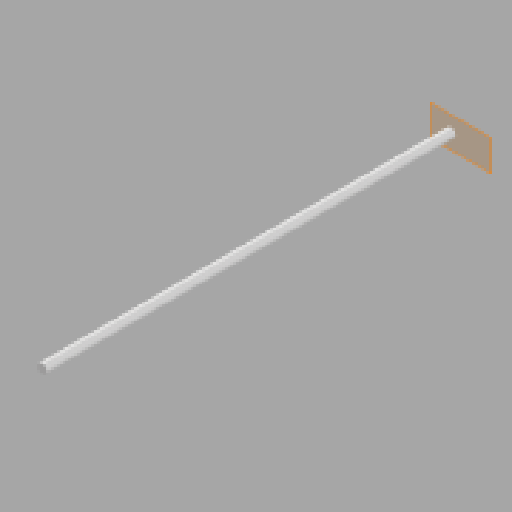
# Autodesk Inventor part: Boom
Saved by Autodesk Inventor 2025 (Build 290162000, 162)
## iProperties
Created: 2025-02-17
Part Number: Boom
Material: Generic
Document SubType Name: Modeling
Designer: Cupri
Density: 1 g/cm^3
Appearance: Default
Mass: 566.296 g
Surface Area: 901.939 cm^2
Volume: 566.296 cm^3
Author: Cupri
Autodesk Inventor part; units mm, degrees
ref_plane "YZ Plane" through (0, 0, 0) normal (1, 0, 0) x (0, 1, 0)
ref_plane "XZ Plane" through (0, 0, 0) normal (0, 1, 0) x (-1, 0, 0)
ref_plane "XY Plane" through (0, 0, 0) normal (0, 0, 1) x (1, 0, 0)
ref_plane "Work Plane1" through (-126.6026, 0, -25.4) normal (0, 0, 1) x (1, 0, 0)
sketch "Sketch1" plane through (-126.6026, 0, -25.4) normal (0, 0, 1) x (1, 0, 0)
  line L0 (132.9264, 43.6548) -> (133.0414, -19.8451) projected
  line L1 (126.6026, 0) -> (-138.4982, 0) construction
  circle A0 centre (-101.9974, 0) radius 12.7
  dimension "d0" = 25.4
  dimension "d1" = 228.6
  constraints: 2 end point, 1 centre point, 1 horizontal, 1 point on line
  measures "d0" diameter of A0
  measures "d1" distance of L1.start A0.centre
extrude "Extrusion1" add sketch "Sketch1" along normal blind 1117.6
body "Solid1"
